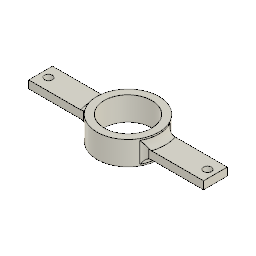
fan-mounter v2 (Autodesk Fusion 360 design; units mm, degrees)
Autodesk Fusion 360 part; units mm, degrees
note: some values were not read from the file. Chosen so that the rebuilt part matches the saved one: which pieces of a blend or face edit are solid. Set by a fixed rule: which sketch regions a step uses.
sketch "スケッチ1" plane through (0, 0, 0) normal (0, 0, 1) x (1, 0, 0)
  circle A0 centre (0, 0) radius 3
  circle A1 centre (0, 0) radius 3.9
  circle A2 centre (-10, 0) radius 0.5
  circle A3 centre (10, 0) radius 0.5
  line L0 (-11, 1.5) -> (11, 1.5)
  line L1 (11, -1.5) -> (-11, -1.5)
  line L2 (-11, 1.5) -> (-11, -1.5)
  line L3 (11, -1.5) -> (11, 1.5)
  line L4 (-11, 0) -> (11, 0)
  line L5 (0, 1.5) -> (0, -1.5)
  dimension "d3" = 6
  dimension "d4" = 7.8
  dimension "d5" = 1
  dimension "d8" = 3
  dimension "d16" = 22
  dimension "d17" = 1
  measures "d3" diameter of A0
  measures "d4" diameter of A1
  measures "d5" diameter of A2
  measures "d17" distance of L2
extrude "押し出し1" add sketch "スケッチ1" along normal blind 1 contours A1 A3 L1 L3 L4 | A1 A3 L0 L3 L4 | A1 A2 L0 L2 L4 | A1 A2 L1 L2 L4 makes body 1 at (-8.1167, 1.1443, 0) makes body 2 at (8.1167, 1.1443, 0)
extrude "押し出し2" add sketch "スケッチ1" along normal blind 3 from surface at -1 contours A0 A1 L1 L4 | A0 A1 L0 L4 | A0 A1 L0 | A0 A1 L1 | A0 A1 L0 L4 | A0 A1 L1 L4 bodies 1 2
fillet "フィレット1" radius 0.8 8 edges at (3.9, 0, 1) (3.9, 0, 0) (3.6, -1.5, 0.5) (3.6, 1.5, 0.5) (-3.9, 0, 1) (-3.9, 0, 0) (-3.6, -1.5, 0.5) (-3.6, 1.5, 0.5) on bodies 1
